Autodesk Inventor part; units mm, degrees
(part 2 of 2)
sketch "circuit" plane through (0, 0, 0) normal (0, 0, 1) x (1, 0, 0)
  line L0 (-16, -10) -> (-12, -15) construction
  line L1 (-16, -15) -> (-12, -10) construction
  line L2 (16, 10) -> (12, 15) construction
  line L3 (16, 15) -> (12, 10) construction
  line L4 (18, 15) -> (-18, -15) construction
  line L5 (-16, -15) -> (-16, 15) construction
  line L6 (16, -15) -> (16, 15) construction
  line L7 (12, -10) -> (12, -15) construction
  line L8 (16, -10) -> (12, -15) construction
  line L9 (-18, 10) -> (18, 10) construction
  line L10 (-18, 15) -> (18, 15) construction
  line L11 (-18, -15) -> (-18, 15) construction
  line L12 (-18, 15) -> (18, -15) construction
  line L13 (-18, -12.5) -> (18, -12.5) construction
  line L14 (18, -15) -> (-18, -15) construction
  line L15 (-18, -10) -> (18, -10) construction
  line L16 (18, 15) -> (18, -15) construction
  circle A0 centre (14, -12.5) radius 0.8 construction
  line L17 (16, -15) -> (12, -10) construction
  line L18 (-12, -10) -> (-12, -15) construction
  circle A1 centre (-14, -12.5) radius 0.8 construction
  line L19 (0, 0) -> (0, 1) construction
  line L20 (0, 0) -> (1, 0) construction
  circle A2 centre (0, 0) radius 15 construction
  line L21 (-12, 10) -> (-12, 15) construction
  circle A3 centre (-14, 12.5) radius 0.8 construction
  line L22 (-16, 10) -> (-12, 15) construction
  line L23 (-16, 15) -> (-12, 10) construction
  line L24 (12, 10) -> (12, 15) construction
  line L25 (-18, 12.5) -> (18, 12.5) construction
  circle A4 centre (14, 12.5) radius 0.8 construction
  line L26 (0, 0) -> (0, 1) construction
  line L27 (16, 15) -> (12, 10) construction
  line L28 (0, 0) -> (1, 0) construction
  line L29 (12, -10) -> (12, -15) construction
  line L30 (-18, -10) -> (18, -10) construction
  line L31 (-16, -10) -> (-12, -15) construction
  circle A5 centre (14, 12.5) radius 0.8 construction
  circle A6 centre (-14, -12.5) radius 0.8 construction
  line L32 (-16, -15) -> (-12, -10) construction
  circle A7 centre (14, -12.5) radius 0.8 construction
  line L33 (16, -15) -> (12, -10) construction
  line L34 (16, -10) -> (12, -15) construction
  line L35 (12, 10) -> (12, 15) construction
  line L36 (16, 10) -> (12, 15) construction
  circle A8 centre (0, 0) radius 7.5 construction
  line L37 (-12, -10) -> (-12, -15) construction
  line L38 (18, 15) -> (18, -15) construction
  line L39 (16, -15) -> (16, 15) construction
  line L40 (-18, -12.5) -> (18, -12.5) construction
  line L41 (18, -15) -> (-18, -15) construction
  circle A9 centre (0, 0) radius 15 construction
  line L42 (-16, -15) -> (-16, 15) construction
  line L43 (-18, 15) -> (18, -15) construction
  line L44 (-18, -15) -> (-18, 15) construction
  line L45 (18, 15) -> (-18, -15) construction
  line L46 (-18, 15) -> (18, 15) construction
  circle A10 centre (-14, 12.5) radius 0.8 construction
  line L47 (-16, 10) -> (-12, 15) construction
  line L48 (-12, 10) -> (-12, 15) construction
  line L49 (-16, 15) -> (-12, 10) construction
  line L50 (-18, 10) -> (18, 10) construction
  line L51 (-18, 12.5) -> (18, 12.5) construction
  line L52 (18, 15) -> (18, -15) construction
  line L53 (18, 15) -> (18, -15) construction
  line L54 (-16, -15) -> (-12, -10) construction
  line L55 (-18, 15) -> (18, 15) construction
  line L56 (-18, 15) -> (18, 15) construction
  line L57 (-16, -15) -> (-16, 15) construction
  line L58 (-16, -15) -> (-16, 15) construction
  line L59 (0, 0) -> (0, 1) construction
  line L60 (-16, 10) -> (-12, 15) construction
  line L61 (-16, 15) -> (-12, 10) construction
  line L62 (18, 15) -> (-18, -15) construction
  line L63 (18, 15) -> (-18, -15) construction
  line L64 (-18, -15) -> (-18, 15) construction
  line L65 (-18, -15) -> (-18, 15) construction
  circle A11 centre (-14, 12.5) radius 0.8 construction
  line L66 (-18, 10) -> (18, 10) construction
  line L67 (-18, 10) -> (18, 10) construction
  line L68 (0, 0) -> (1, 0) construction
  circle A12 centre (0, 0) radius 15 construction
  line L69 (0, 0) -> (1, 0) construction
  circle A13 centre (0, 0) radius 7.5 construction
  circle A14 centre (0, 0) radius 15 construction
  line L70 (16, 15) -> (12, 10) construction
  circle A15 centre (14, 12.5) radius 0.8 construction
  line L71 (16, 15) -> (12, 10) construction
  line L72 (16, -15) -> (16, 15) construction
  line L73 (16, -15) -> (16, 15) construction
  line L74 (-12, 10) -> (-12, 15) construction
  line L75 (-12, 10) -> (-12, 15) construction
  line L76 (12, 10) -> (12, 15) construction
  line L77 (16, 10) -> (12, 15) construction
  line L78 (-18, 12.5) -> (18, 12.5) construction
  line L79 (-18, -10) -> (18, -10) construction
  line L80 (-18, -12.5) -> (18, -12.5) construction
  line L81 (-18, 15) -> (18, -15) construction
  circle A16 centre (-14, 12.5) radius 0.8 construction
  line L82 (-16, 10) -> (-12, 15) construction
  line L83 (-16, 15) -> (-12, 10) construction
  line L84 (-12, -10) -> (-12, -15) construction
  line L85 (12, 10) -> (12, 15) construction
  line L86 (16, 10) -> (12, 15) construction
  line L87 (-18, 12.5) -> (18, 12.5) construction
  line L88 (-18, -12.5) -> (18, -12.5) construction
  line L89 (-18, 15) -> (18, -15) construction
  circle A17 centre (-14, -12.5) radius 0.8 construction
  circle A18 centre (-14, -12.5) radius 0.8 construction
  circle A19 centre (-14, -12.5) radius 1 projected
  line L90 (-16, -10) -> (-12, -15) construction
  line L91 (-16, -10) -> (-12, -15) construction
  line L92 (-16, -15) -> (-12, -10) construction
  line L93 (-6.8217, -17.6764) -> (6.8217, -17.6764) projected
  line L94 (-18, -10) -> (18, -10) construction
  line L95 (-12, -10) -> (-12, -15) construction
  line L96 (18, 8.5) -> (18, -8.5) projected
  circle A20 centre (14, -12.5) radius 0.8 construction
  line L97 (16, -15) -> (12, -10) construction
  circle A21 centre (14, -12.5) radius 0.8 construction
  circle A22 centre (14, -12.5) radius 1 projected
  line L98 (16, -15) -> (12, -10) construction
  line L99 (12, -10) -> (12, -15) construction
  line L100 (16, -10) -> (12, -15) construction
  line L101 (16, -10) -> (12, -15) construction
  line L102 (18, -15) -> (-18, -15) construction
  line L103 (18, -15) -> (-18, -15) construction
  line L104 (12, -10) -> (12, -15) construction
  circle A23 centre (0, 0) radius 7.5 projected
  line L105 (0, 0) -> (0, 1) construction
  line L106 (-18, 8.5) -> (-18, -8.5) projected
  circle A24 centre (14, 12.5) radius 0.8 construction
  circle A25 centre (14, 12.5) radius 1 projected
  circle A26 centre (-14, 12.5) radius 1 projected
  line L107 (0, 127.2792) -> (0, -127.2792) construction
  line L108 (-84, 120) -> (29.25, 40.7015) construction
  line L109 (-25.25, 18.5) -> (-80.9717, 292.3807) construction
  line L110 (-25.3613, 19.2922) -> (-65.8646, 307.4878) construction
  line L111 (-25.25, 18.5) -> (-47.5722, 302.1307) construction
  line L112 (-29.25, 45.5846) -> (-29.75, 45.2345) construction
  line L113 (13.7445, 51.5585) -> (13.2857, 50.9032) construction
  line L114 (84, 120) -> (-29.25, 40.7015) construction
  line L115 (29.25, 55) -> (29.75, 55) construction
  line L116 (29.75, 55) -> (29.75, -30) construction
  line L117 (-29.75, 55) -> (-29.75, -30) construction
  line L118 (-25.25, 55) -> (-25.25, -30) construction
  line L119 (9.0748, 50.5556) -> (14.3993, 46.8274) construction
  line L120 (11.6554, 51.1902) -> (14.1129, 49.4694) construction
  line L121 (9.6483, 51.3748) -> (14.9728, 47.6465) construction
  line L122 (13.7445, 51.5585) -> (13.0892, 52.0174) construction
  line L123 (14.1129, 49.4694) -> (15.8336, 51.9269) construction
  line L124 (11.6554, 51.1902) -> (15.8336, 51.9269) construction
  line L125 (13.3762, 53.6476) -> (11.6554, 51.1902) construction
  line L126 (13.3762, 53.6476) -> (14.1129, 49.4694) construction
  line L127 (15.8336, 51.9269) -> (13.3762, 53.6476) construction
  line L128 (14.3993, 46.8274) -> (18.4143, 52.5615) construction
  line L129 (9.0748, 50.5556) -> (18.4143, 52.5615) construction
  line L130 (13.0898, 56.2897) -> (9.0748, 50.5556) construction
  line L131 (13.0898, 56.2897) -> (14.3993, 46.8274) construction
  line L132 (12.5162, 55.4705) -> (17.8407, 51.7423) construction
  line L133 (18.4143, 52.5615) -> (13.0898, 56.2897) construction
  circle A27 centre (13.7445, 51.5585) radius 0.8 construction
  line L134 (-29.25, 55) -> (29.25, 55) construction
  line L135 (-1.8558, 55) -> (-29.25, 35.8184) construction
  line L136 (29.25, 11.5) -> (29.25, 55) construction
  line L137 (-8.9966, 50) -> (8.9966, 50) construction
  line L138 (1.8558, 55) -> (29.25, 35.8184) construction
  line L139 (-11.6554, 51.1902) -> (-14.1129, 49.4694) construction
  line L140 (-29.25, 11.5) -> (-29.25, 55) construction
  line L141 (-13.7445, 51.5585) -> (-13.2857, 50.9032) construction
  line L142 (-13.3762, 53.6476) -> (-14.1129, 49.4694) construction
  line L143 (-13.0898, 56.2897) -> (-14.3993, 46.8274) construction
  line L144 (-9.0748, 50.5556) -> (-14.3993, 46.8274) construction
  line L145 (-9.6483, 51.3748) -> (-14.9728, 47.6465) construction
  line L146 (-14.1129, 49.4694) -> (-15.8336, 51.9269) construction
  line L147 (-14.3993, 46.8274) -> (-18.4143, 52.5615) construction
  line L148 (-13.3762, 53.6476) -> (-11.6554, 51.1902) construction
  line L149 (-15.8336, 51.9269) -> (-13.3762, 53.6476) construction
  line L150 (-12.5162, 55.4705) -> (-17.8407, 51.7423) construction
  line L151 (-13.0898, 56.2897) -> (-9.0748, 50.5556) construction
  line L152 (-18.4143, 52.5615) -> (-13.0898, 56.2897) construction
  line L153 (-15.8034, 55) -> (-29.25, 45.5846) construction
  line L154 (-29.25, 55) -> (-29.75, 55) construction
  line L155 (-13.7445, 51.5585) -> (-13.0892, 52.0174) construction
  circle A28 centre (-13.7445, 51.5585) radius 0.8 construction
  line L156 (-11.6554, 51.1902) -> (-15.8336, 51.9269) construction
  line L157 (-9.0748, 50.5556) -> (-18.4143, 52.5615) construction
  line L158 (-14.1129, 49.4694) -> (-15.8336, 51.9269) construction
  line L159 (-29.25, 55) -> (-29.75, 55) construction
  line L160 (29.25, 55) -> (29.75, 55) construction
  line L161 (8.8296, 55) -> (15.8034, 55) projected
  line L162 (-8.9966, 50) -> (8.9966, 50) projected
  line L163 (13.3762, 53.6476) -> (15.8336, 51.9269) projected
  line L164 (23.7807, 49.4143) -> (15.8034, 55) projected
  line L165 (14.1129, 49.4694) -> (11.6554, 51.1902) projected
  line L166 (15.8336, 51.9269) -> (14.1129, 49.4694) projected
  line L167 (8.9966, 50) -> (16.3936, 44.8205) projected
  line L168 (19.3049, 42.7821) -> (21.2944, 33.4219) projected
  line L169 (23.7807, 49.4143) -> (29.75, 21.3308) projected
  line L170 (16.3936, 44.8205) -> (0, 28.4269) projected
  line L171 (19.3049, 42.7821) -> (2.1213, 25.5985) projected
  line L172 (11.6554, 51.1902) -> (13.3762, 53.6476) projected
  circle A29 centre (-13.7445, 51.5585) radius 0.8 construction
  line L173 (-15.8336, 51.9269) -> (-13.3762, 53.6476) construction
  line L174 (-29.25, 45.5846) -> (-29.75, 45.2345) construction
  line L175 (-13.3762, 53.6476) -> (-14.1129, 49.4694) construction
  line L176 (-11.6554, 51.1902) -> (-15.8336, 51.9269) construction
  line L177 (-13.3762, 53.6476) -> (-11.6554, 51.1902) construction
  line L178 (-11.6554, 51.1902) -> (-14.1129, 49.4694) construction
  line L179 (-14.3993, 46.8274) -> (-18.4143, 52.5615) construction
  line L180 (-13.0898, 56.2897) -> (-9.0748, 50.5556) construction
  line L181 (-9.0748, 50.5556) -> (-14.3993, 46.8274) construction
  line L182 (-1.8558, 55) -> (-29.25, 35.8184) construction
  line L183 (-29.25, 11.5) -> (-29.25, 55) construction
  line L184 (29.75, 55) -> (29.75, -30) construction
  line L185 (-29.75, 55) -> (-29.75, -30) construction
  line L186 (29.25, 11.5) -> (29.25, 55) construction
  line L187 (1.8558, 55) -> (29.25, 35.8184) construction
  line L188 (-29.25, 55) -> (29.25, 55) construction
  line L189 (-15.8034, 55) -> (-29.25, 45.5846) construction
  line L190 (-8.9966, 50) -> (8.9966, 50) construction
  line L191 (-9.6483, 51.3748) -> (-14.9728, 47.6465) construction
  line L192 (-13.7445, 51.5585) -> (-13.2857, 50.9032) construction
  line L193 (-13.7445, 51.5585) -> (-13.0892, 52.0174) construction
  line L194 (-9.0748, 50.5556) -> (-18.4143, 52.5615) construction
  line L195 (-12.5162, 55.4705) -> (-17.8407, 51.7423) construction
  line L196 (-18.4143, 52.5615) -> (-13.0898, 56.2897) construction
  line L197 (-13.0898, 56.2897) -> (-14.3993, 46.8274) construction
  line L198 (-15.8034, 55) -> (-8.8296, 55) projected
  line L199 (-29.75, 45.2345) -> (-29.25, 45.5846) projected
  line L200 (-23.7807, 49.4143) -> (-15.8034, 55) projected
  line L201 (-16.3936, 44.8205) -> (-8.9966, 50) projected
  line L202 (-19.3049, 42.7821) -> (-21.2944, 33.4219) projected
  line L203 (-23.7807, 49.4143) -> (-29.75, 21.3308) projected
  line L204 (-15.8336, 51.9269) -> (-14.1129, 49.4694) projected
  line L205 (-13.3762, 53.6476) -> (-15.8336, 51.9269) projected
  line L206 (-11.6554, 51.1902) -> (-13.3762, 53.6476) projected
  line L207 (-14.1129, 49.4694) -> (-11.6554, 51.1902) projected
  line L208 (-16.3936, 44.8205) -> (0, 28.4269) projected
  line L209 (-19.3049, 42.7821) -> (-2.1213, 25.5985) projected
  line L210 (84, 120) -> (-29.25, 40.7015) construction
  line L211 (-8.8296, 55) -> (8.8296, 55) projected
  line L212 (-84, 120) -> (29.25, 40.7015) construction
  line L213 (-29.75, -30) -> (29.75, -30) construction
  line L214 (-29.25, -11.5) -> (-29.25, 11.5) construction
  line L215 (-18, 11.5) -> (-29.25, -11.5) construction
  line L216 (-29.25, 11.5) -> (-18, -11.5) construction
  line L217 (-90, -90) -> (90, 90) construction
  line L218 (-90, 90) -> (90, -90) construction
  line L219 (18, 11.5) -> (29.25, -11.5) construction
  line L220 (29.25, 11.5) -> (18, -11.5) construction
  line L221 (29.25, -11.5) -> (29.25, 11.5) construction
  line L222 (29.25, 11.5) -> (18, 11.5) construction
  line L223 (-29.25, 11.5) -> (-18, 11.5) construction
  line L224 (29.25, 11.5) -> (18, -11.5) construction
  line L225 (18, 11.5) -> (29.25, -11.5) construction
  line L226 (29.25, -11.5) -> (29.25, 11.5) construction
  line L227 (-90, -90) -> (90, 90) construction
  line L228 (-90, 90) -> (90, -90) construction
  line L229 (-18, 11.5) -> (-29.25, -11.5) construction
  line L230 (29.25, 11.5) -> (18, 11.5) construction
  line L231 (-29.25, 11.5) -> (-18, 11.5) construction
  line L232 (-29.25, -11.5) -> (-29.25, 11.5) construction
  line L233 (-29.25, 11.5) -> (-18, -11.5) construction
  line L234 (29.25, -11.5) -> (29.25, 11.5) construction
  line L235 (29.25, -11.5) -> (29.25, 11.5) construction
  line L236 (18, 11.5) -> (29.25, -11.5) construction
  line L237 (18, 11.5) -> (29.25, -11.5) construction
  line L238 (29.25, 11.5) -> (18, 11.5) construction
  line L239 (29.25, 11.5) -> (18, -11.5) construction
  line L240 (29.25, 11.5) -> (18, 11.5) construction
  line L241 (29.25, 11.5) -> (18, -11.5) construction
  line L242 (-18, 11.5) -> (-29.25, -11.5) construction
  line L243 (-18, 11.5) -> (-29.25, -11.5) construction
  line L244 (-29.25, 11.5) -> (-18, -11.5) construction
  line L245 (-29.25, 11.5) -> (-18, -11.5) construction
  line L246 (-29.25, -11.5) -> (-29.25, 11.5) construction
  line L247 (-29.25, -11.5) -> (-29.25, 11.5) construction
  line L248 (-90, 90) -> (90, -90) construction
  line L249 (-90, 90) -> (90, -90) construction
  line L250 (-90, -90) -> (90, 90) construction
  line L251 (-90, -90) -> (90, 90) construction
  line L252 (29.75, 21.3308) -> (29.75, 8.5) projected
  line L253 (-29.75, 21.3308) -> (-29.75, 8.5) projected
  line L254 (-29.25, 11.5) -> (-18, 11.5) construction
  line L255 (-29.25, 11.5) -> (-18, 11.5) construction
  line L256 (-18, -11.5) -> (-29.25, -11.5) construction
  line L257 (18, -11.5) -> (29.25, -11.5) construction
  line L258 (18, -11.5) -> (29.25, -11.5) construction
  line L259 (-18, -11.5) -> (-29.25, -11.5) construction
  line L260 (18, -11.5) -> (29.25, -11.5) construction
  line L261 (18, -11.5) -> (29.25, -11.5) construction
  line L262 (29.75, -8.5) -> (22.3317, -30) projected
  line L263 (-18, -11.5) -> (-29.25, -11.5) construction
  line L264 (-29.75, -8.5) -> (-22.3317, -30) projected
  line L265 (-18, -11.5) -> (-29.25, -11.5) construction
  line L266 (-29.75, 8.5) -> (29.75, 8.5) construction
  line L267 (-29.75, -8.5) -> (29.75, -8.5) construction
  line L268 (-127.2792, 0) -> (127.2792, 0) construction
  line L269 (-15.6458, 54.5) -> (-23.3325, 49.1177)
  line L270 (-23.3325, 49.1177) -> (-24.3995, 44.0978)
  line L271 (-24.3995, 44.0978) -> (-18.9665, 44.0978)
  line L272 (-18.9665, 44.0978) -> (-8.3787, 49.1177)
  line L273 (-8.3787, 49.1177) -> (0, 48.4722)
  line L274 (-15.6458, 54.5) -> (0, 54.5)
  line L275 (15.6458, 54.5) -> (23.3325, 49.1177)
  line L276 (23.3325, 49.1177) -> (24.3995, 44.0978)
  line L277 (24.3995, 44.0978) -> (18.9665, 44.0978)
  line L278 (18.9665, 44.0978) -> (8.3787, 49.1177)
  line L279 (8.3787, 49.1177) -> (0, 48.4722)
  line L280 (15.6458, 54.5) -> (0, 54.5)
  line L281 (-28.8719, 19.2922) -> (-14.6507, 21.4093)
  line L282 (-28.8719, 19.2922) -> (-27.8681, 12.5498)
  line L283 (-27.8681, 12.5498) -> (-24.1381, 10.5882)
  line L284 (-24.1381, 10.5882) -> (-15.1785, 7.6027)
  line L285 (-15.1785, 7.6027) -> (-11.6554, -10.6244)
  line L286 (-11.6554, -10.6244) -> (-11.3888, -14.0123)
  line L287 (-11.3888, -14.0123) -> (-9.9476, -16.8873)
  line L288 (-9.9476, -16.8873) -> (0, -16.4077)
  line L289 (-14.6507, 21.4093) -> (0, 19.2922)
  line L290 (28.8719, 19.2922) -> (14.6507, 21.4093)
  line L291 (28.8719, 19.2922) -> (27.8681, 12.5498)
  line L292 (27.8681, 12.5498) -> (24.1381, 10.5882)
  line L293 (24.1381, 10.5882) -> (15.1785, 7.6027)
  line L294 (15.1785, 7.6027) -> (11.6554, -10.6244)
  line L295 (11.6554, -10.6244) -> (11.3888, -14.0123)
  line L296 (11.3888, -14.0123) -> (9.9476, -16.8873)
  line L297 (9.9476, -16.8873) -> (0, -16.4077)
  line L298 (14.6507, 21.4093) -> (0, 19.2922)
  circle A30 centre (0, 0) radius 4.35
  point P0 (0, 0)
  point P1 (13.256, 24.3963)
  point P2 (-13.256, 24.3963)
  point P3 (11.0823, 53.4227)
  point P4 (-11.0823, 53.4227)
  point P5 (-8.8296, 55)
  point P6 (-8.8296, 55)
  point P7 (-11.0823, 53.4227)
  dimension "d387" = 0.5
  dimension "d388" = 0.5
  dimension "d389" = 0.5
  dimension "d393" = 8.7
  constraints: 60 end point, 13 horizontal alignment, 2 horizontal, 2 parallel, 1 centre point, 124 other
  measures "d387" distance between parallel lines of L153 L269
  measures "d388" distance between parallel lines of L203 L270
  measures "d393" diameter of A30
extrude "押し出し1" add sketch "スケッチ5" against normal blind 1 contours L282 L281 L235 L233 L236 L245 L244 L283 L284 L240 L242 L241 L261 L260 L259 L231 L232 L230 | L268 L267 L266 L265 | L277 L278 L279 L280 | L301 L302 L303 L285 | L288 L287 L286 | L289 L290 L291 | L304 L305 L306 L307
extrude "押し出し2" cut sketch "スケッチ5" against normal blind 1 contours L268 L267 L266 L265 | L277 L278 L279 L280
extrude "押し出し4" cut sketch "スケッチ5" against normal blind 1 contours L288 L287 L286 | L289 L290 L291
extrude "押し出し5" cut sketch "スケッチ5" against normal blind 0.1 contours L301 L302 L303 L285 | L304 L305 L306 L307
ref_plane "作業平面1" through (0, 0, 4) normal (0, 0, 1) x (1, 0, 0)
sketch "スケッチ8" plane through (0, 0, 4) normal (0, 0, 1) x (1, 0, 0)
  line L0 (-24.3995, 44.0978) -> (-18.9665, 44.0978) projected
  line L1 (-18.9665, 44.0978) -> (-8.3787, 49.1177) projected
  line L2 (-8.3787, 49.1177) -> (0, 48.4722) projected
  line L3 (8.3787, 49.1177) -> (0, 48.4722) projected
  line L4 (18.9665, 44.0978) -> (8.3787, 49.1177) projected
  line L5 (24.3995, 44.0978) -> (18.9665, 44.0978) projected
  line L6 (23.3325, 49.1177) -> (24.3995, 44.0978) projected
  line L7 (15.6458, 54.5) -> (23.3325, 49.1177) projected
  line L8 (15.6458, 54.5) -> (0, 54.5) projected
  line L9 (-15.6458, 54.5) -> (0, 54.5) projected
  line L10 (-15.6458, 54.5) -> (-23.3325, 49.1177) projected
  line L11 (-23.3325, 49.1177) -> (-24.3995, 44.0978) projected
  line L12 (-28.8719, 19.2922) -> (-27.8681, 12.5498) projected
  line L13 (-28.8719, 19.2922) -> (-14.6507, 21.4093) projected
  line L14 (-14.6507, 21.4093) -> (0, 19.2922) projected
  line L15 (14.6507, 21.4093) -> (0, 19.2922) projected
  line L16 (28.8719, 19.2922) -> (14.6507, 21.4093) projected
  line L17 (28.8719, 19.2922) -> (27.8681, 12.5498) projected
  line L18 (27.8681, 12.5498) -> (24.1381, 10.5882) projected
  line L19 (24.1381, 10.5882) -> (15.1785, 7.6027) projected
  line L20 (15.1785, 7.6027) -> (11.6554, -10.6244) projected
  line L21 (11.6554, -10.6244) -> (11.3888, -14.0123) projected
  line L22 (11.3888, -14.0123) -> (9.9476, -16.8873) projected
  line L23 (17.4751, 17.0681) -> (18.1709, 22.0195) projected
  line L24 (18.1709, 22.0195) -> (28.0736, 20.6277) projected
  line L25 (28.0736, 20.6277) -> (27.3777, 15.6764) projected
  line L26 (27.3777, 15.6764) -> (17.4751, 17.0681) projected
  line L27 (-27.3777, 15.6764) -> (-28.0736, 20.6277) projected
  line L28 (-28.0736, 20.6277) -> (-18.1709, 22.0195) projected
  line L29 (-18.1709, 22.0195) -> (-17.4751, 17.0681) projected
  line L30 (-17.4751, 17.0681) -> (-27.3777, 15.6764) projected
  line L31 (25.6517, -13.5042) -> (23.113, -20.862) projected
  line L32 (23.113, -20.862) -> (16.8015, -17.6162) projected
  line L33 (16.8015, -17.6162) -> (25.6517, -13.5042) projected
  line L34 (-25.6517, -13.5042) -> (-16.8015, -17.6162) projected
  line L35 (-16.8015, -17.6162) -> (-23.113, -20.862) projected
  line L36 (-23.113, -20.862) -> (-25.6517, -13.5042) projected
  line L37 (15.8336, 51.9269) -> (14.1129, 49.4694) projected
  line L38 (14.1129, 49.4694) -> (11.6554, 51.1902) projected
  line L39 (11.6554, 51.1902) -> (13.3762, 53.6476) projected
  line L40 (13.3762, 53.6476) -> (15.8336, 51.9269) projected
  line L41 (-11.6554, 51.1902) -> (-14.1129, 49.4694) projected
  line L42 (-14.1129, 49.4694) -> (-15.8336, 51.9269) projected
  line L43 (-15.8336, 51.9269) -> (-13.3762, 53.6476) projected
  line L44 (-13.3762, 53.6476) -> (-11.6554, 51.1902) projected
  line L45 (-29.75, 21.3308) -> (-29.75, 8.5) projected
  line L46 (-29.75, 8.5) -> (-18, 8.5) projected
  line L47 (-18, 8.5) -> (-18, -8.5) projected
  line L48 (-18, -8.5) -> (-29.75, -8.5) projected
  line L49 (-29.75, -8.5) -> (-22.3317, -30) projected
  line L50 (-22.3317, -30) -> (22.3317, -30) projected
  line L51 (22.3317, -30) -> (29.75, -8.5) projected
  line L52 (29.75, -8.5) -> (18, -8.5) projected
  line L53 (18, -8.5) -> (18, 8.5) projected
  line L54 (18, 8.5) -> (29.75, 8.5) projected
  line L55 (29.75, 8.5) -> (29.75, 21.3308) projected
  line L56 (29.75, 21.3308) -> (23.7807, 49.4143) projected
  line L57 (23.7807, 49.4143) -> (15.8034, 55) projected
  line L58 (15.8034, 55) -> (-15.8034, 55) projected
  line L59 (-15.8034, 55) -> (-23.7807, 49.4143) projected
  line L60 (-23.7807, 49.4143) -> (-29.75, 21.3308) projected
  circle A0 centre (0, 0) radius 7.5 projected
  circle A1 centre (-14, 12.5) radius 1 projected
  circle A2 centre (14, 12.5) radius 1 projected
  circle A3 centre (14, -12.5) radius 1 projected
  circle A4 centre (-14, -12.5) radius 1 projected
  line L61 (-21.4865, -25.218) -> (-6.8217, -17.6764) projected
  line L62 (-6.8217, -17.6764) -> (6.8217, -17.6764) projected
  line L63 (6.8217, -17.6764) -> (21.4865, -25.218) projected
  line L64 (21.4865, -25.218) -> (20.895, -26.9322) projected
  line L65 (20.895, -26.9322) -> (-20.895, -26.9322) projected
  line L66 (-20.895, -26.9322) -> (-21.4865, -25.218) projected
  line L67 (21.2944, 33.4219) -> (13.256, 24.3963) projected
  line L68 (13.256, 24.3963) -> (2.1213, 25.5985) projected
  line L69 (2.1213, 25.5985) -> (19.3049, 42.7821) projected
  line L70 (19.3049, 42.7821) -> (21.2944, 33.4219) projected
  line L71 (-19.3049, 42.7821) -> (-2.1213, 25.5985) projected
  line L72 (-2.1213, 25.5985) -> (-13.256, 24.3963) projected
  line L73 (-13.256, 24.3963) -> (-21.2944, 33.4219) projected
  line L74 (-21.2944, 33.4219) -> (-19.3049, 42.7821) projected
  line L75 (-16.3936, 44.8205) -> (-8.9966, 50) projected
  line L76 (-8.9966, 50) -> (8.9966, 50) projected
  line L77 (8.9966, 50) -> (16.3936, 44.8205) projected
  line L78 (16.3936, 44.8205) -> (0, 28.4269) projected
  line L79 (0, 28.4269) -> (-16.3936, 44.8205) projected
  line L80 (9.9476, -16.8873) -> (0, -16.4077) projected
  line L81 (-9.9476, -16.8873) -> (0, -16.4077) projected
  line L82 (-11.3888, -14.0123) -> (-9.9476, -16.8873) projected
  line L83 (-11.6554, -10.6244) -> (-11.3888, -14.0123) projected
  line L84 (-15.1785, 7.6027) -> (-11.6554, -10.6244) projected
  line L85 (-24.1381, 10.5882) -> (-15.1785, 7.6027) projected
  line L86 (-27.8681, 12.5498) -> (-24.1381, 10.5882) projected
  circle A5 centre (0, 0) radius 4.35 projected
  point P0 (-14.1948, 46.3602)
  point P1 (14.1948, 46.3602)
extrude "押し出し7" add sketch "スケッチ8" along normal blind 0.8 contours L13 L27 L30 L29 L14 L15 L16 L23 L26 L25 L17 L18 L19 L20 L21 L22 L80 L81 L82 L83 L84 L85 L86 L12 | L13 L29 L30 L27 | L16 L25 L26 L23 | A0 | A1 | A2
ref_plane "作業平面2" through (0, 0, 1) normal (0, 0, 1) x (1, 0, 0)
sketch "スケッチ9" plane through (0, 0, 1) normal (0, 0, 1) x (1, 0, 0)
  line L0 (-23.3325, 49.1177) -> (-24.3995, 44.0978) projected
  line L1 (-24.3995, 44.0978) -> (-18.9665, 44.0978) projected
  line L2 (-18.9665, 44.0978) -> (-8.3787, 49.1177) projected
  line L3 (-8.3787, 49.1177) -> (0, 48.4722) projected
  line L4 (8.3787, 49.1177) -> (0, 48.4722) projected
  line L5 (18.9665, 44.0978) -> (8.3787, 49.1177) projected
  line L6 (24.3995, 44.0978) -> (18.9665, 44.0978) projected
  line L7 (23.3325, 49.1177) -> (24.3995, 44.0978) projected
  line L8 (15.6458, 54.5) -> (23.3325, 49.1177) projected
  line L9 (15.6458, 54.5) -> (0, 54.5) projected
  line L10 (-15.6458, 54.5) -> (0, 54.5) projected
  line L11 (17.4751, 17.0681) -> (18.1709, 22.0195) projected
  line L12 (18.1709, 22.0195) -> (28.0736, 20.6277) projected
  line L13 (28.0736, 20.6277) -> (27.3777, 15.6764) projected
  line L14 (27.3777, 15.6764) -> (17.4751, 17.0681) projected
  line L15 (-27.3777, 15.6764) -> (-28.0736, 20.6277) projected
  line L16 (-28.0736, 20.6277) -> (-18.1709, 22.0195) projected
  line L17 (-18.1709, 22.0195) -> (-17.4751, 17.0681) projected
  line L18 (-17.4751, 17.0681) -> (-27.3777, 15.6764) projected
  line L19 (25.6517, -13.5042) -> (23.113, -20.862) projected
  line L20 (23.113, -20.862) -> (16.8015, -17.6162) projected
  line L21 (16.8015, -17.6162) -> (25.6517, -13.5042) projected
  line L22 (-25.6517, -13.5042) -> (-16.8015, -17.6162) projected
  line L23 (-16.8015, -17.6162) -> (-23.113, -20.862) projected
  line L24 (-23.113, -20.862) -> (-25.6517, -13.5042) projected
  line L25 (15.8336, 51.9269) -> (14.1129, 49.4694) projected
  line L26 (14.1129, 49.4694) -> (11.6554, 51.1902) projected
  line L27 (11.6554, 51.1902) -> (13.3762, 53.6476) projected
  line L28 (13.3762, 53.6476) -> (15.8336, 51.9269) projected
  line L29 (-11.6554, 51.1902) -> (-14.1129, 49.4694) projected
  line L30 (-14.1129, 49.4694) -> (-15.8336, 51.9269) projected
  line L31 (-15.8336, 51.9269) -> (-13.3762, 53.6476) projected
  line L32 (-13.3762, 53.6476) -> (-11.6554, 51.1902) projected
  line L33 (-29.75, 21.3308) -> (-29.75, 8.5) projected
  line L34 (-29.75, 8.5) -> (-18, 8.5) projected
  line L35 (-18, 8.5) -> (-18, -8.5) projected
  line L36 (-18, -8.5) -> (-29.75, -8.5) projected
  line L37 (-29.75, -8.5) -> (-22.3317, -30) projected
  line L38 (-22.3317, -30) -> (22.3317, -30) projected
  line L39 (22.3317, -30) -> (29.75, -8.5) projected
  line L40 (29.75, -8.5) -> (18, -8.5) projected
  line L41 (18, -8.5) -> (18, 8.5) projected
  line L42 (18, 8.5) -> (29.75, 8.5) projected
  line L43 (29.75, 8.5) -> (29.75, 21.3308) projected
  line L44 (29.75, 21.3308) -> (23.7807, 49.4143) projected
  line L45 (23.7807, 49.4143) -> (15.8034, 55) projected
  line L46 (15.8034, 55) -> (-15.8034, 55) projected
  line L47 (-15.8034, 55) -> (-23.7807, 49.4143) projected
  line L48 (-23.7807, 49.4143) -> (-29.75, 21.3308) projected
  circle A0 centre (0, 0) radius 7.5 projected
  circle A1 centre (-14, 12.5) radius 1 projected
  circle A2 centre (14, 12.5) radius 1 projected
  circle A3 centre (14, -12.5) radius 1 projected
  circle A4 centre (-14, -12.5) radius 1 projected
  line L49 (-21.4865, -25.218) -> (-6.8217, -17.6764) projected
  line L50 (-6.8217, -17.6764) -> (6.8217, -17.6764) projected
  line L51 (6.8217, -17.6764) -> (21.4865, -25.218) projected
  line L52 (21.4865, -25.218) -> (20.895, -26.9322) projected
  line L53 (20.895, -26.9322) -> (-20.895, -26.9322) projected
  line L54 (-20.895, -26.9322) -> (-21.4865, -25.218) projected
  line L55 (21.2944, 33.4219) -> (13.256, 24.3963) projected
  line L56 (13.256, 24.3963) -> (2.1213, 25.5985) projected
  line L57 (2.1213, 25.5985) -> (19.3049, 42.7821) projected
  line L58 (19.3049, 42.7821) -> (21.2944, 33.4219) projected
  line L59 (-19.3049, 42.7821) -> (-2.1213, 25.5985) projected
  line L60 (-2.1213, 25.5985) -> (-13.256, 24.3963) projected
  line L61 (-13.256, 24.3963) -> (-21.2944, 33.4219) projected
  line L62 (-21.2944, 33.4219) -> (-19.3049, 42.7821) projected
  line L63 (-16.3936, 44.8205) -> (-8.9966, 50) projected
  line L64 (-8.9966, 50) -> (8.9966, 50) projected
  line L65 (8.9966, 50) -> (16.3936, 44.8205) projected
  line L66 (16.3936, 44.8205) -> (0, 28.4269) projected
  line L67 (0, 28.4269) -> (-16.3936, 44.8205) projected
  line L68 (-15.6458, 54.5) -> (-23.3325, 49.1177) projected
extrude "押し出し8" add sketch "スケッチ9" along normal blind 0.4 contours L68 L10 L9 L8 L7 L6 L5 L65 L64 L63 L2 L1 L0 | L63 L64 L65 L5 L4 L3 L2
